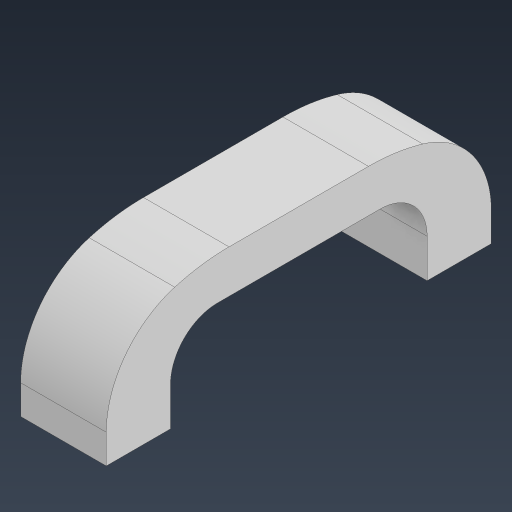
# Autodesk Inventor part: Raczka
Saved by Autodesk Inventor 2024 (Build 280153000, 153)
## iProperties
Created: 2023-12-20
Part Number: Raczka
Material: Generic
Document SubType Name: Modeling
Designer: Piter
Density: 1 g/cm^3
Appearance: Default
Author: Piter
Autodesk Inventor part; units mm, degrees
ref_plane "YZ Plane" through (0, 0, 0) normal (1, 0, 0) x (0, 1, 0)
ref_plane "XZ Plane" through (0, 0, 0) normal (0, 1, 0) x (-1, 0, 0)
ref_plane "XY Plane" through (0, 0, 0) normal (0, 0, 1) x (1, 0, 0)
sketch "Sketch1" plane through (0, 0, 0) normal (1, 0, 0) x (0, 1, 0)
  line L0 (0, 0) -> (0, 30)
  line L1 (0, 30) -> (20, 30)
  line L2 (20, 30) -> (20, -60)
  line L3 (20, -60) -> (0, -60)
  line L4 (0, -60) -> (0, 30)
  line L5 (20, 30) -> (30, 30)
  line L6 (30, 30) -> (30, -30)
  line L7 (30, -30) -> (20, -30)
  line L8 (20, -30) -> (20, 30)
  line L9 (0, 30) -> (20, 30)
  line L10 (20, 30) -> (20, 45)
  line L11 (20, 45) -> (0, 45)
  line L12 (0, 45) -> (0, 30)
  line L13 (20, 0) -> (0, 0)
  line L14 (0, -60) -> (20, -30)
  line L15 (20, -30) -> (30, -30)
  line L16 (0, -60) -> (20, -30)
  line L17 (20, -30) -> (20, -45)
  line L18 (20, -45) -> (0, -45)
  line L19 (0, -45) -> (0, -60)
  line L20 (20, 45) -> (30, 30)
  line L21 (30, -30) -> (20, -45)
  line L22 (20, -30) -> (0, -30)
  point P0 (20, -30)
  point P1 (20, -30)
  point P2 (20, -30)
  point P3 (10, -45)
  point P4 (20, -30)
  point P5 (0, -45)
  point P6 (10, -45)
  dimension "d0" = 30
  dimension "d1" = 20
  dimension "d2" = 90
  dimension "d3" = 10
  dimension "d4" = 20
  dimension "d5" = 15
  constraints: 46 end point, 6 parallel, 5 perpendicular, 3 horizontal, 3 symmetric about line, 1 midpoint, 1 point on line, 1 vertical
  measures "d0" distance of L0.start L0.end
  measures "d1" distance of L2.end L3.end
  measures "d2" distance of L1.end L2.end
  measures "d3" distance of L6.end L7.end
  measures "d4" distance of L11.end L10.end
  measures "d5" distance of L10.end L9.end
extrude "Extrusion1" add sketch "Sketch1" along normal blind 20 contours L12 L11 L10 L1 | L22 L14 L18 L4 | L2 L5 L6 L7 | L10 L20 L5 | L7 L21 L2 | L2 L18 L14
fillet "Fillet2" radius 45.25 2 edges at (10, 30, -30) (10, 30, 30)
fillet "Fillet3" radius 11 2 edges at (10, 20, 30) (10, 20, -30)
fillet "Fillet4" radius 22.25 2 edges at (10, 20, -45) (10, 20, 45)
sketch "Sketch3" plane through (0, 0, -45) normal (0, -1, 0) x (1, 0, 0)
  circle A0 centre (14, 7.5) radius 3.25
  line L0 (0, 0) -> (20, 0) projected
  circle A1 centre (6, 7.5) radius 1
  line L1 (0, 45) -> (21.3664, 45)
  circle A2 centre (14, 82.5) radius 3.25
  circle A3 centre (6, 82.5) radius 1
  line L2 (20, 15) -> (20, 0) projected
  line L3 (0, 15) -> (0, 0) projected
  point P0 (20, 90)
  point P1 (20, 7.5)
  dimension "d21" = 6.5
  dimension "d22" = 7.5
  dimension "d23" = 2
  dimension "d28" = 7.5
  dimension "d29" = 6
  dimension "d30" = 6
  constraints: 4 centre point, 3 symmetric about line, 2 end point, 1 horizontal, 1 midpoint, 2 other
  measures "d21" diameter of A0
  measures "d22" distance from line of A0.centre L0
  measures "d23" diameter of A1
  measures "d28" distance from line of L0 A1.centre
  measures "d29" distance of point (20, 7.5) A0.centre
  measures "d30" distance from line of L3 A1.centre
extrude "Extrusion4" cut sketch "Sketch3" against normal blind 3.5 contours A0 | A2
extrude "Extrusion5" cut sketch "Sketch3" against normal blind 10 contours A1 | A3
body "Solid1"
